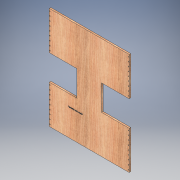
# Autodesk Inventor part: Placeholder Belly Pan
Saved by Autodesk Inventor 2018 (Build 220112000, 112)
## iProperties
Created: 2020-01-18
Part Number: Placeholder Belly Pan
Material: Wood (Birch)
Document SubType Name: Modeling
Designer: maste
Density: 0.55 g/cm^3
Appearance: Birch - Natural Polished
Author: maste
Autodesk Inventor part; units mm, degrees
ref_plane "YZ Plane" through (0, 0, 0) normal (1, 0, 0) x (0, 1, 0)
ref_plane "XZ Plane" through (0, 0, 0) normal (0, 1, 0) x (-1, 0, 0)
ref_plane "XY Plane" through (0, 0, 0) normal (0, 0, 1) x (1, 0, 0)
sketch "Sketch1" plane through (0, 0, 0) normal (0, 0, 1) x (1, 0, 0)
  line L0 (0, 0) -> (476.25, 0)
  line L1 (476.25, 0) -> (476.25, 228.6)
  line L2 (476.25, 228.6) -> (311.15, 228.6)
  line L3 (311.15, 228.6) -> (311.15, 381)
  line L4 (311.15, 381) -> (476.25, 381)
  line L5 (476.25, 381) -> (476.25, 609.6)
  line L6 (476.25, 609.6) -> (0, 609.6)
  line L7 (0, 609.6) -> (0, 381)
  line L8 (0, 381) -> (165.1, 381)
  line L9 (165.1, 381) -> (165.1, 228.6)
  line L10 (165.1, 228.6) -> (0, 228.6)
  line L11 (0, 228.6) -> (0, 0)
  dimension "d0" = 476.25
  dimension "d1" = 228.6
  dimension "d2" = 165.1
  dimension "d3" = 152.4
  dimension "d4" = 228.6
  dimension "d5" = 165.1
  constraints: 24 end point, 8 perpendicular, 7 point on line, 1 horizontal
  measures "d0" distance of L0.start L0.end
  measures "d1" distance of L0.end L1.end
  measures "d2" distance of L1.end L2.end
  measures "d3" distance of L2.end L3.end
  measures "d4" distance of L4.end L5.end
  measures "d5" distance of L7.end L8.end
extrude "Extrusion1" add sketch "Sketch1" along normal blind 9.525
sketch "Sketch2" plane through (0, 0, 9.525) normal (0, 0, 1) x (1, 0, 0)
  line L0 (0, 0) -> (3.175, 0) construction
  line L1 (0, 0) -> (476.25, 0) construction
  line L2 (3.175, 0) -> (3.175, 12.7) construction
  line L3 (3.175, 12.7) -> (3.175, 38.1) construction
  line L4 (3.175, 38.1) -> (3.175, 63.5) construction
  line L5 (3.175, 63.5) -> (3.175, 88.9) construction
  line L6 (3.175, 88.9) -> (3.175, 114.3) construction
  line L7 (3.175, 114.3) -> (3.175, 139.7) construction
  line L8 (3.175, 139.7) -> (3.175, 165.1) construction
  line L9 (3.175, 165.1) -> (3.175, 190.5) construction
  line L10 (3.175, 190.5) -> (3.175, 215.9) construction
  circle A0 centre (3.175, 12.7) radius 2.5797
  circle A1 centre (3.175, 38.1) radius 2.5797
  circle A2 centre (3.175, 63.5) radius 2.5797
  circle A3 centre (3.175, 88.9) radius 2.5797
  circle A4 centre (3.175, 114.3) radius 2.5797
  circle A5 centre (3.175, 139.7) radius 2.5797
  circle A6 centre (3.175, 165.1) radius 2.5797
  circle A7 centre (3.175, 190.5) radius 2.5797
  circle A8 centre (3.175, 215.9) radius 2.5797
  line L11 (238.125, 0) -> (238.125, 609.6) construction
  line L12 (476.25, 609.6) -> (0, 609.6) construction
  line L13 (0, 304.8) -> (476.25, 304.8) construction
  line L14 (473.075, 0) -> (473.075, 12.7) construction
  line L15 (473.075, 12.7) -> (473.075, 38.1) construction
  line L16 (473.075, 38.1) -> (473.075, 63.5) construction
  line L17 (473.075, 63.5) -> (473.075, 88.9) construction
  line L18 (473.075, 88.9) -> (473.075, 114.3) construction
  line L19 (473.075, 114.3) -> (473.075, 139.7) construction
  line L20 (473.075, 139.7) -> (473.075, 165.1) construction
  line L21 (473.075, 165.1) -> (473.075, 190.5) construction
  line L22 (473.075, 190.5) -> (473.075, 215.9) construction
  circle A9 centre (473.075, 12.7) radius 2.5797
  circle A10 centre (473.075, 38.1) radius 2.5797
  circle A11 centre (473.075, 63.5) radius 2.5797
  circle A12 centre (473.075, 88.9) radius 2.5797
  circle A13 centre (473.075, 114.3) radius 2.5797
  circle A14 centre (473.075, 139.7) radius 2.5797
  circle A15 centre (473.075, 165.1) radius 2.5797
  circle A16 centre (473.075, 190.5) radius 2.5797
  circle A17 centre (473.075, 215.9) radius 2.5797
  line L23 (0, 609.6) -> (3.175, 609.6) construction
  line L24 (0, 609.6) -> (476.25, 609.6) construction
  line L25 (3.175, 609.6) -> (3.175, 596.9) construction
  line L26 (3.175, 596.9) -> (3.175, 571.5) construction
  line L27 (3.175, 571.5) -> (3.175, 546.1) construction
  line L28 (3.175, 546.1) -> (3.175, 520.7) construction
  line L29 (3.175, 520.7) -> (3.175, 495.3) construction
  line L30 (3.175, 495.3) -> (3.175, 469.9) construction
  line L31 (3.175, 469.9) -> (3.175, 444.5) construction
  line L32 (3.175, 444.5) -> (3.175, 419.1) construction
  line L33 (3.175, 419.1) -> (3.175, 393.7) construction
  circle A18 centre (3.175, 596.9) radius 2.5797
  circle A19 centre (3.175, 571.5) radius 2.5797
  circle A20 centre (3.175, 546.1) radius 2.5797
  circle A21 centre (3.175, 520.7) radius 2.5797
  circle A22 centre (3.175, 495.3) radius 2.5797
  circle A23 centre (3.175, 469.9) radius 2.5797
  circle A24 centre (3.175, 444.5) radius 2.5797
  circle A25 centre (3.175, 419.1) radius 2.5797
  circle A26 centre (3.175, 393.7) radius 2.5797
  line L34 (473.075, 495.3) -> (473.075, 469.9) construction
  circle A27 centre (473.075, 495.3) radius 2.5797
  line L35 (473.075, 520.7) -> (473.075, 495.3) construction
  line L36 (473.075, 546.1) -> (473.075, 520.7) construction
  line L37 (473.075, 571.5) -> (473.075, 546.1) construction
  line L38 (473.075, 596.9) -> (473.075, 571.5) construction
  circle A28 centre (473.075, 596.9) radius 2.5797
  line L39 (473.075, 609.6) -> (473.075, 596.9) construction
  circle A29 centre (473.075, 520.7) radius 2.5797
  circle A30 centre (473.075, 469.9) radius 2.5797
  circle A31 centre (473.075, 444.5) radius 2.5797
  line L40 (473.075, 444.5) -> (473.075, 419.1) construction
  circle A32 centre (473.075, 419.1) radius 2.5797
  line L41 (473.075, 419.1) -> (473.075, 393.7) construction
  circle A33 centre (473.075, 393.7) radius 2.5797
  circle A34 centre (473.075, 571.5) radius 2.5797
  circle A35 centre (473.075, 546.1) radius 2.5797
  line L42 (473.075, 469.9) -> (473.075, 444.5) construction
  dimension "d8" = 3.175
  dimension "d9" = 12.7
  dimension "d10" = 25.4
  dimension "d11" = 25.4
  dimension "d12" = 25.4
  dimension "d13" = 25.4
  dimension "d14" = 25.4
  dimension "d15" = 25.4
  dimension "d16" = 25.4
  dimension "d17" = 25.4
  dimension "d18" = 5.1594
  constraints: 82 end point, 57 symmetric about line, 36 centre point, 36 coincident, 30 point on line, 2 midpoint, 2 vertical, 1 horizontal, 27 other
  measures "d8" distance of L0.start L0.end
  measures "d9" distance of L0.end L2.end
  measures "d10" distance of L2.end L3.end
  measures "d11" distance of L3.end L4.end
  measures "d12" distance of L4.end L5.end
  measures "d13" distance of L5.end L6.end
  measures "d14" distance of L6.end L7.end
  measures "d15" distance of L7.end L8.end
  measures "d16" distance of L8.end L9.end
  measures "d17" distance of L9.end L10.end
  measures "d18" diameter of A0
extrude "Extrusion2" cut sketch "Sketch2" against normal blind 82.55
sketch "Sketch3" plane through (0, 0, 9.525) normal (0, 0, 1) x (1, 0, 0)
  line L0 (113.0988, 164.0574) -> (392.0139, 164.0574) construction
  line L1 (392.0139, 164.0574) -> (392.0139, 75.3899) construction
  line L2 (392.0139, 75.3899) -> (113.0988, 75.3899) construction
  line L3 (113.0988, 75.3899) -> (113.0988, 164.0574) construction
  line L4 (117.2238, 161.3206) -> (116.957, 160.871)
  line L5 (116.957, 160.871) -> (115.6183, 161.7602)
  line L6 (115.6183, 161.7602) -> (115.6479, 160.2684)
  line L7 (115.6479, 160.2684) -> (115.1341, 160.2684)
  line L8 (115.1341, 160.2684) -> (115.1588, 161.7602)
  line L9 (115.1588, 161.7602) -> (113.83, 160.8661)
  line L10 (113.83, 160.8661) -> (113.5583, 161.3156)
  line L11 (113.5583, 161.3156) -> (115.0057, 162.1653)
  line L12 (115.0057, 162.1653) -> (113.5583, 163.0101)
  line L13 (113.5583, 163.0101) -> (113.83, 163.4596)
  line L14 (113.83, 163.4596) -> (115.1638, 162.5655)
  line L15 (115.1638, 162.5655) -> (115.1341, 164.0574)
  line L16 (115.1341, 164.0574) -> (115.6479, 164.0574)
  line L17 (115.6479, 164.0574) -> (115.6133, 162.5655)
  line L18 (115.6133, 162.5655) -> (116.957, 163.4547)
  line L19 (116.957, 163.4547) -> (117.2238, 163.0051)
  line L20 (117.2238, 163.0051) -> (115.7763, 162.1653)
  line L21 (115.7763, 162.1653) -> (117.2238, 161.3206)
  spline S0 degree 2 poles (122.065, 160.1004) (122.065, 158.9543) (120.9733, 157.6007) (120.1384, 157.6007) knots 0 0 0 1 2 2 2
  spline S1 degree 2 poles (120.1384, 157.6007) (119.7975, 157.6007) (119.2739, 157.7588) (119.0022, 157.9218) knots 0 0 0 1 2 2 2
  line L22 (119.0022, 157.9218) -> (119.0022, 156.0051)
  line L23 (119.0022, 156.0051) -> (118.2315, 156.0051)
  line L24 (118.2315, 156.0051) -> (118.2315, 162.2641)
  line L25 (118.2315, 162.2641) -> (119.0022, 162.2641)
  line L26 (119.0022, 162.2641) -> (119.0022, 161.7849)
  spline S2 degree 2 poles (119.0022, 161.7849) (119.2887, 162.0468) (119.9902, 162.3926) (120.4002, 162.3926) knots 0 0 0 1 2 2 2
  spline S3 degree 2 poles (120.4002, 162.3926) (121.1857, 162.3926) (122.065, 161.1477) (122.065, 160.1004) knots 0 0 0 1 2 2 2
  spline S4 degree 2 poles (121.2697, 160.0115) (121.2697, 160.7969) (120.7707, 161.6614) (120.2125, 161.6614) knots 0 0 0 1 2 2 2
  spline S5 degree 2 poles (120.2125, 161.6614) (119.8864, 161.6614) (119.2739, 161.37) (119.0022, 161.1427) knots 0 0 0 1 2 2 2
  line L27 (119.0022, 161.1427) -> (119.0022, 158.5443)
  spline S6 degree 2 poles (119.0022, 158.5443) (119.3035, 158.401) (119.7333, 158.2923) (120.0099, 158.2923) knots 0 0 0 1 2 2 2
  spline S7 degree 2 poles (120.0099, 158.2923) (120.6077, 158.2923) (121.2697, 159.1717) (121.2697, 160.0115) knots 0 0 0 1 2 2 2
  line L28 (125.2908, 161.4391) -> (125.2513, 161.4391)
  spline S8 degree 2 poles (125.2513, 161.4391) (125.1624, 161.4638) (124.9697, 161.4737) (124.8364, 161.4737) knots 0 0 0 1 2 2 2
  spline S9 degree 2 poles (124.8364, 161.4737) (124.5251, 161.4737) (123.9126, 161.202) (123.6359, 160.9353) knots 0 0 0 1 2 2 2
  line L29 (123.6359, 160.9353) -> (123.6359, 157.6897)
  line L30 (123.6359, 157.6897) -> (122.8653, 157.6897)
  line L31 (122.8653, 157.6897) -> (122.8653, 162.2641)
  line L32 (122.8653, 162.2641) -> (123.6359, 162.2641)
  line L33 (123.6359, 162.2641) -> (123.6359, 161.5824)
  spline S10 degree 2 poles (123.6359, 161.5824) (124.0558, 161.9578) (124.6832, 162.2641) (124.9796, 162.2641) knots 0 0 0 1 2 2 2
  spline S11 degree 2 poles (124.9796, 162.2641) (125.0982, 162.2641) (125.2167, 162.2542) (125.2908, 162.2394) knots 0 0 0 1 2 2 2
  line L34 (125.2908, 162.2394) -> (125.2908, 161.4391)
  spline S12 degree 2 poles (129.648, 159.9769) (129.648, 158.8209) (128.5364, 157.5612) (127.6077, 157.5612) knots 0 0 0 1 2 2 2
  spline S13 degree 2 poles (127.6077, 157.5612) (126.6543, 157.5612) (125.5625, 158.8604) (125.5625, 159.9769) knots 0 0 0 1 2 2 2
  spline S14 degree 2 poles (125.5625, 159.9769) (125.5625, 161.123) (126.6889, 162.3926) (127.6077, 162.3926) knots 0 0 0 1 2 2 2
  spline S15 degree 2 poles (127.6077, 162.3926) (128.5364, 162.3926) (129.648, 161.1279) (129.648, 159.9769) knots 0 0 0 1 2 2 2
  spline S16 degree 2 poles (128.8526, 159.9769) (128.8526, 160.8661) (128.2055, 161.7306) (127.6077, 161.7306) knots 0 0 0 1 2 2 2
  spline S17 degree 2 poles (127.6077, 161.7306) (127.01, 161.7306) (126.3579, 160.8661) (126.3579, 159.9769) knots 0 0 0 1 2 2 2
  spline S18 degree 2 poles (126.3579, 159.9769) (126.3579, 159.1124) (127.01, 158.2232) (127.6077, 158.2232) knots 0 0 0 1 2 2 2
  spline S19 degree 2 poles (127.6077, 158.2232) (128.2005, 158.2232) (128.8526, 159.0976) (128.8526, 159.9769) knots 0 0 0 1 2 2 2
  spline S20 degree 2 poles (134.2718, 160.051) (134.2718, 158.9296) (133.185, 157.5612) (132.365, 157.5612) knots 0 0 0 1 2 2 2
  spline S21 degree 2 poles (132.365, 157.5612) (131.9945, 157.5612) (131.4659, 157.744) (131.209, 157.9021) knots 0 0 0 1 2 2 2
  line L35 (131.209, 157.9021) -> (131.1596, 157.6897)
  line L36 (131.1596, 157.6897) -> (130.4384, 157.6897)
  line L37 (130.4384, 157.6897) -> (130.4384, 164.0574)
  line L38 (130.4384, 164.0574) -> (131.209, 164.0574)
  line L39 (131.209, 164.0574) -> (131.209, 161.7849)
  spline S22 degree 2 poles (131.209, 161.7849) (131.5005, 162.0468) (132.1772, 162.3926) (132.607, 162.3926) knots 0 0 0 1 2 2 2
  spline S23 degree 2 poles (132.607, 162.3926) (133.3826, 162.3926) (134.2718, 161.1526) (134.2718, 160.051) knots 0 0 0 1 2 2 2
  spline S24 degree 2 poles (133.4765, 159.9917) (133.4765, 160.8118) (132.9775, 161.6614) (132.4243, 161.6614) knots 0 0 0 1 2 2 2
  spline S25 degree 2 poles (132.4243, 161.6614) (132.113, 161.6614) (131.4708, 161.365) (131.209, 161.1378) knots 0 0 0 1 2 2 2
  line L40 (131.209, 161.1378) -> (131.209, 158.5146)
  spline S26 degree 2 poles (131.209, 158.5146) (131.5005, 158.3714) (131.95, 158.2528) (132.2168, 158.2528) knots 0 0 0 1 2 2 2
  spline S27 degree 2 poles (132.2168, 158.2528) (132.8046, 158.2528) (133.4765, 159.0877) (133.4765, 159.9917) knots 0 0 0 1 2 2 2
  spline S28 degree 2 poles (137.6212, 158.1738) (137.5273, 158.1046) (137.2111, 157.8576) (137.0629, 157.7835) knots 0 0 0 1 2 2 2
  spline S29 degree 2 poles (137.0629, 157.7835) (136.8604, 157.6748) (136.48, 157.5612) (136.1342, 157.5612) knots 0 0 0 1 2 2 2
  spline S30 degree 2 poles (136.1342, 157.5612) (135.8526, 157.5612) (135.3438, 157.7736) (135.1511, 157.9663) knots 0 0 0 1 2 2 2
  spline S31 degree 2 poles (135.1511, 157.9663) (134.9684, 158.154) (134.7461, 158.7073) (134.7461, 159.0136) knots 0 0 0 1 2 2 2
  spline S32 degree 2 poles (134.7461, 159.0136) (134.7461, 159.4878) (135.1462, 160.1597) (135.5809, 160.3523) knots 0 0 0 1 2 2 2
  spline S33 degree 2 poles (135.5809, 160.3523) (135.9663, 160.5302) (137.0135, 160.6636) (137.6212, 160.6981) knots 0 0 0 1 2 2 2
  line L41 (137.6212, 160.6981) -> (137.6212, 160.8463)
  spline S34 degree 2 poles (137.6212, 160.8463) (137.6212, 161.1131) (137.4581, 161.4441) (137.3099, 161.5379) knots 0 0 0 1 2 2 2
  spline S35 degree 2 poles (137.3099, 161.5379) (137.1617, 161.6318) (136.7369, 161.6911) (136.5097, 161.6911) knots 0 0 0 1 2 2 2
  spline S36 degree 2 poles (136.5097, 161.6911) (136.2429, 161.6911) (135.5217, 161.533) (135.161, 161.3799) knots 0 0 0 1 2 2 2
  line L42 (135.161, 161.3799) -> (135.1166, 161.3799)
  line L43 (135.1166, 161.3799) -> (135.1166, 162.1653)
  spline S37 degree 2 poles (135.1166, 162.1653) (135.329, 162.2246) (136.1243, 162.3728) (136.5146, 162.3728) knots 0 0 0 1 2 2 2
  spline S38 degree 2 poles (136.5146, 162.3728) (136.9888, 162.3728) (137.636, 162.2246) (137.8929, 162.0319) knots 0 0 0 1 2 2 2
  spline S39 degree 2 poles (137.8929, 162.0319) (138.1448, 161.8442) (138.3918, 161.2465) (138.3918, 160.8167) knots 0 0 0 1 2 2 2
  line L44 (138.3918, 160.8167) -> (138.3918, 157.6897)
  line L45 (138.3918, 157.6897) -> (137.6212, 157.6897)
  line L46 (137.6212, 157.6897) -> (137.6212, 158.1738)
  line L47 (137.6212, 158.816) -> (137.6212, 160.0856)
  spline S40 degree 2 poles (137.6212, 160.0856) (137.3445, 160.0609) (136.5097, 159.9769) (136.2478, 159.8978) knots 0 0 0 1 2 2 2
  spline S41 degree 2 poles (136.2478, 159.8978) (135.9416, 159.804) (135.5414, 159.4137) (135.5414, 159.0679) knots 0 0 0 1 2 2 2
  spline S42 degree 2 poles (135.5414, 159.0679) (135.5414, 158.6727) (135.986, 158.2726) (136.4109, 158.2726) knots 0 0 0 1 2 2 2
  spline S43 degree 2 poles (136.4109, 158.2726) (136.7715, 158.2726) (137.3643, 158.5838) (137.6212, 158.816) knots 0 0 0 1 2 2 2
  spline S44 degree 2 poles (143.3071, 160.051) (143.3071, 158.9296) (142.2203, 157.5612) (141.4003, 157.5612) knots 0 0 0 1 2 2 2
  spline S45 degree 2 poles (141.4003, 157.5612) (141.0298, 157.5612) (140.5012, 157.744) (140.2443, 157.9021) knots 0 0 0 1 2 2 2
  line L48 (140.2443, 157.9021) -> (140.1949, 157.6897)
  line L49 (140.1949, 157.6897) -> (139.4737, 157.6897)
  line L50 (139.4737, 157.6897) -> (139.4737, 164.0574)
  line L51 (139.4737, 164.0574) -> (140.2443, 164.0574)
  line L52 (140.2443, 164.0574) -> (140.2443, 161.7849)
  spline S46 degree 2 poles (140.2443, 161.7849) (140.5358, 162.0468) (141.2126, 162.3926) (141.6424, 162.3926) knots 0 0 0 1 2 2 2
  spline S47 degree 2 poles (141.6424, 162.3926) (142.4179, 162.3926) (143.3071, 161.1526) (143.3071, 160.051) knots 0 0 0 1 2 2 2
  spline S48 degree 2 poles (142.5118, 159.9917) (142.5118, 160.8118) (142.0129, 161.6614) (141.4596, 161.6614) knots 0 0 0 1 2 2 2
  spline S49 degree 2 poles (141.4596, 161.6614) (141.1483, 161.6614) (140.5061, 161.365) (140.2443, 161.1378) knots 0 0 0 1 2 2 2
  line L53 (140.2443, 161.1378) -> (140.2443, 158.5146)
  spline S50 degree 2 poles (140.2443, 158.5146) (140.5358, 158.3714) (140.9853, 158.2528) (141.2521, 158.2528) knots 0 0 0 1 2 2 2
  spline S51 degree 2 poles (141.2521, 158.2528) (141.84, 158.2528) (142.5118, 159.0877) (142.5118, 159.9917) knots 0 0 0 1 2 2 2
  line L54 (144.8929, 157.6897) -> (144.1222, 157.6897)
  line L55 (144.1222, 157.6897) -> (144.1222, 164.0574)
  line L56 (144.1222, 164.0574) -> (144.8929, 164.0574)
  line L57 (144.8929, 164.0574) -> (144.8929, 157.6897)
  line L58 (149.6156, 162.2641) -> (147.1554, 156.0051)
  line L59 (147.1554, 156.0051) -> (146.3304, 156.0051)
  line L60 (146.3304, 156.0051) -> (147.1505, 157.912)
  line L61 (147.1505, 157.912) -> (145.4906, 162.2641)
  line L62 (145.4906, 162.2641) -> (146.3206, 162.2641)
  line L63 (146.3206, 162.2641) -> (147.5704, 158.8753)
  line L64 (147.5704, 158.8753) -> (148.8153, 162.2641)
  line L65 (148.8153, 162.2641) -> (149.6156, 162.2641)
  line L66 (156.4081, 157.6897) -> (155.6375, 157.6897)
  line L67 (155.6375, 157.6897) -> (155.6375, 160.298)
  spline S52 degree 2 poles (155.6375, 160.298) (155.6375, 160.6142) (155.5782, 161.1576) (155.4893, 161.3206) knots 0 0 0 1 2 2 2
  spline S53 degree 2 poles (155.4893, 161.3206) (155.3954, 161.4935) (155.0595, 161.6614) (154.773, 161.6614) knots 0 0 0 1 2 2 2
  spline S54 degree 2 poles (154.773, 161.6614) (154.4864, 161.6614) (153.8788, 161.3552) (153.5873, 161.1082) knots 0 0 0 1 2 2 2
  line L68 (153.5873, 161.1082) -> (153.5873, 157.6897)
  line L69 (153.5873, 157.6897) -> (152.8167, 157.6897)
  line L70 (152.8167, 157.6897) -> (152.8167, 162.2641)
  line L71 (152.8167, 162.2641) -> (153.5873, 162.2641)
  line L72 (153.5873, 162.2641) -> (153.5873, 161.7553)
  spline S55 degree 2 poles (153.5873, 161.7553) (153.9332, 162.0665) (154.6001, 162.3926) (154.9755, 162.3926) knots 0 0 0 1 2 2 2
  spline S56 degree 2 poles (154.9755, 162.3926) (155.6473, 162.3926) (156.4081, 161.5034) (156.4081, 160.6586) knots 0 0 0 1 2 2 2
  line L73 (156.4081, 160.6586) -> (156.4081, 157.6897)
  spline S57 degree 2 poles (161.2493, 159.9769) (161.2493, 158.8209) (160.1378, 157.5612) (159.2091, 157.5612) knots 0 0 0 1 2 2 2
  spline S58 degree 2 poles (159.2091, 157.5612) (158.2557, 157.5612) (157.1639, 158.8604) (157.1639, 159.9769) knots 0 0 0 1 2 2 2
  spline S59 degree 2 poles (157.1639, 159.9769) (157.1639, 161.123) (158.2903, 162.3926) (159.2091, 162.3926) knots 0 0 0 1 2 2 2
  spline S60 degree 2 poles (159.2091, 162.3926) (160.1378, 162.3926) (161.2493, 161.1279) (161.2493, 159.9769) knots 0 0 0 1 2 2 2
  spline S61 degree 2 poles (160.454, 159.9769) (160.454, 160.8661) (159.8069, 161.7306) (159.2091, 161.7306) knots 0 0 0 1 2 2 2
  spline S62 degree 2 poles (159.2091, 161.7306) (158.6114, 161.7306) (157.9593, 160.8661) (157.9593, 159.9769) knots 0 0 0 1 2 2 2
  spline S63 degree 2 poles (157.9593, 159.9769) (157.9593, 159.1124) (158.6114, 158.2232) (159.2091, 158.2232) knots 0 0 0 1 2 2 2
  spline S64 degree 2 poles (159.2091, 158.2232) (159.8019, 158.2232) (160.454, 159.0976) (160.454, 159.9769) knots 0 0 0 1 2 2 2
  spline S65 degree 2 poles (163.423, 157.6007) (162.7956, 157.6007) (162.0891, 158.317) (162.0891, 159.0926) knots 0 0 0 1 2 2 2
  line L74 (162.0891, 159.0926) -> (162.0891, 161.6269)
  line L75 (162.0891, 161.6269) -> (161.5704, 161.6269)
  line L76 (161.5704, 161.6269) -> (161.5704, 162.2641)
  line L77 (161.5704, 162.2641) -> (162.0891, 162.2641)
  line L78 (162.0891, 162.2641) -> (162.0891, 163.5782)
  line L79 (162.0891, 163.5782) -> (162.8598, 163.5782)
  line L80 (162.8598, 163.5782) -> (162.8598, 162.2641)
  line L81 (162.8598, 162.2641) -> (164.2776, 162.2641)
  line L82 (164.2776, 162.2641) -> (164.2776, 161.6269)
  line L83 (164.2776, 161.6269) -> (162.8598, 161.6269)
  line L84 (162.8598, 161.6269) -> (162.8598, 159.4483)
  spline S66 degree 2 poles (162.8598, 159.4483) (162.8598, 159.1025) (162.8845, 158.7221) (162.9685, 158.5591) knots 0 0 0 1 2 2 2
  spline S67 degree 2 poles (162.9685, 158.5591) (163.0376, 158.4158) (163.3489, 158.2726) (163.6156, 158.2726) knots 0 0 0 1 2 2 2
  spline S68 degree 2 poles (163.6156, 158.2726) (163.8033, 158.2726) (164.1541, 158.3862) (164.2331, 158.4208) knots 0 0 0 1 2 2 2
  line L85 (164.2331, 158.4208) -> (164.2776, 158.4208)
  line L86 (164.2776, 158.4208) -> (164.2776, 157.7292)
  spline S69 degree 2 poles (164.2776, 157.7292) (164.0602, 157.6699) (163.6156, 157.6007) (163.423, 157.6007) knots 0 0 0 1 2 2 2
  spline S70 degree 2 poles (168.8471, 157.6007) (168.2197, 157.6007) (167.5133, 158.317) (167.5133, 159.0926) knots 0 0 0 1 2 2 2
  line L87 (167.5133, 159.0926) -> (167.5133, 161.6269)
  line L88 (167.5133, 161.6269) -> (166.9946, 161.6269)
  line L89 (166.9946, 161.6269) -> (166.9946, 162.2641)
  line L90 (166.9946, 162.2641) -> (167.5133, 162.2641)
  line L91 (167.5133, 162.2641) -> (167.5133, 163.5782)
  line L92 (167.5133, 163.5782) -> (168.2839, 163.5782)
  line L93 (168.2839, 163.5782) -> (168.2839, 162.2641)
  line L94 (168.2839, 162.2641) -> (169.7017, 162.2641)
  line L95 (169.7017, 162.2641) -> (169.7017, 161.6269)
  line L96 (169.7017, 161.6269) -> (168.2839, 161.6269)
  line L97 (168.2839, 161.6269) -> (168.2839, 159.4483)
  spline S71 degree 2 poles (168.2839, 159.4483) (168.2839, 159.1025) (168.3086, 158.7221) (168.3926, 158.5591) knots 0 0 0 1 2 2 2
  spline S72 degree 2 poles (168.3926, 158.5591) (168.4618, 158.4158) (168.773, 158.2726) (169.0398, 158.2726) knots 0 0 0 1 2 2 2
  spline S73 degree 2 poles (169.0398, 158.2726) (169.2275, 158.2726) (169.5782, 158.3862) (169.6573, 158.4208) knots 0 0 0 1 2 2 2
  line L98 (169.6573, 158.4208) -> (169.7017, 158.4208)
  line L99 (169.7017, 158.4208) -> (169.7017, 157.7292)
  spline S74 degree 2 poles (169.7017, 157.7292) (169.4844, 157.6699) (169.0398, 157.6007) (168.8471, 157.6007) knots 0 0 0 1 2 2 2
  spline S75 degree 2 poles (174.0292, 159.9769) (174.0292, 158.8209) (172.9177, 157.5612) (171.989, 157.5612) knots 0 0 0 1 2 2 2
  spline S76 degree 2 poles (171.989, 157.5612) (171.0355, 157.5612) (169.9438, 158.8604) (169.9438, 159.9769) knots 0 0 0 1 2 2 2
  spline S77 degree 2 poles (169.9438, 159.9769) (169.9438, 161.123) (171.0701, 162.3926) (171.989, 162.3926) knots 0 0 0 1 2 2 2
  spline S78 degree 2 poles (171.989, 162.3926) (172.9177, 162.3926) (174.0292, 161.1279) (174.0292, 159.9769) knots 0 0 0 1 2 2 2
  spline S79 degree 2 poles (173.2339, 159.9769) (173.2339, 160.8661) (172.5867, 161.7306) (171.989, 161.7306) knots 0 0 0 1 2 2 2
  spline S80 degree 2 poles (171.989, 161.7306) (171.3912, 161.7306) (170.7391, 160.8661) (170.7391, 159.9769) knots 0 0 0 1 2 2 2
  spline S81 degree 2 poles (170.7391, 159.9769) (170.7391, 159.1124) (171.3912, 158.2232) (171.989, 158.2232) knots 0 0 0 1 2 2 2
  spline S82 degree 2 poles (171.989, 158.2232) (172.5818, 158.2232) (173.2339, 159.0976) (173.2339, 159.9769) knots 0 0 0 1 2 2 2
  spline S83 degree 2 poles (178.6728, 157.581) (178.2134, 157.581) (177.4181, 157.828) (177.1562, 157.9663) knots 0 0 0 1 2 2 2
  line L100 (177.1562, 157.9663) -> (177.1562, 158.8308)
  line L101 (177.1562, 158.8308) -> (177.1958, 158.8308)
  spline S84 degree 2 poles (177.1958, 158.8308) (177.2946, 158.7518) (177.5613, 158.564) (177.7836, 158.4603) knots 0 0 0 1 2 2 2
  spline S85 degree 2 poles (177.7836, 158.4603) (177.9763, 158.3664) (178.4505, 158.2281) (178.7025, 158.2281) knots 0 0 0 1 2 2 2
  spline S86 degree 2 poles (178.7025, 158.2281) (178.8853, 158.2281) (179.3052, 158.3121) (179.404, 158.3813) knots 0 0 0 1 2 2 2
  spline S87 degree 2 poles (179.404, 158.3813) (179.5472, 158.4751) (179.6757, 158.6875) (179.6757, 158.9049) knots 0 0 0 1 2 2 2
  spline S88 degree 2 poles (179.6757, 158.9049) (179.6757, 159.1766) (179.3793, 159.4582) (178.9989, 159.552) knots 0 0 0 1 2 2 2
  spline S89 degree 2 poles (178.9989, 159.552) (178.8507, 159.5866) (178.3764, 159.6854) (178.1739, 159.7398) knots 0 0 0 1 2 2 2
  spline S90 degree 2 poles (178.1739, 159.7398) (177.6502, 159.8929) (177.176, 160.5252) (177.176, 160.9748) knots 0 0 0 1 2 2 2
  spline S91 degree 2 poles (177.176, 160.9748) (177.176, 161.5972) (178.1097, 162.3728) (178.8803, 162.3728) knots 0 0 0 1 2 2 2
  spline S92 degree 2 poles (178.8803, 162.3728) (179.2607, 162.3728) (180.0313, 162.1851) (180.2932, 162.0418) knots 0 0 0 1 2 2 2
  line L102 (180.2932, 162.0418) -> (180.2932, 161.2168)
  line L103 (180.2932, 161.2168) -> (180.2536, 161.2168)
  spline S93 degree 2 poles (180.2536, 161.2168) (179.9572, 161.454) (179.236, 161.7257) (178.8655, 161.7257) knots 0 0 0 1 2 2 2
  spline S94 degree 2 poles (178.8655, 161.7257) (178.4851, 161.7257) (177.9615, 161.4046) (177.9615, 161.0835) knots 0 0 0 1 2 2 2
  spline S95 degree 2 poles (177.9615, 161.0835) (177.9615, 160.792) (178.2727, 160.5104) (178.6185, 160.4215) knots 0 0 0 1 2 2 2
  spline S96 degree 2 poles (178.6185, 160.4215) (178.7865, 160.377) (179.2113, 160.2881) (179.4435, 160.2338) knots 0 0 0 1 2 2 2
  spline S97 degree 2 poles (179.4435, 160.2338) (179.9474, 160.1053) (180.4611, 159.5175) (180.4611, 159.0086) knots 0 0 0 1 2 2 2
  spline S98 degree 2 poles (180.4611, 159.0086) (180.4611, 158.7122) (180.2289, 158.1886) (180.0017, 157.9959) knots 0 0 0 1 2 2 2
  spline S99 degree 2 poles (180.0017, 157.9959) (179.7596, 157.7934) (179.1421, 157.581) (178.6728, 157.581) knots 0 0 0 1 2 2 2
  spline S100 degree 2 poles (182.9954, 157.5859) (182.5211, 157.5859) (181.7357, 157.8774) (181.4541, 158.1738) knots 0 0 0 1 2 2 2
  spline S101 degree 2 poles (181.4541, 158.1738) (181.1725, 158.4652) (180.8613, 159.3643) (180.8613, 159.967) knots 0 0 0 1 2 2 2
  spline S102 degree 2 poles (180.8613, 159.967) (180.8613, 160.5697) (181.1824, 161.449) (181.4541, 161.7454) knots 0 0 0 1 2 2 2
  spline S103 degree 2 poles (181.4541, 161.7454) (181.7258, 162.0468) (182.531, 162.3679) (182.9954, 162.3679) knots 0 0 0 1 2 2 2
  spline S104 degree 2 poles (182.9954, 162.3679) (183.3708, 162.3679) (184.0723, 162.1554) (184.344, 162.0171) knots 0 0 0 1 2 2 2
  line L104 (184.344, 162.0171) -> (184.344, 161.1526)
  line L105 (184.344, 161.1526) -> (184.2995, 161.1526)
  spline S105 degree 2 poles (184.2995, 161.1526) (184.2156, 161.2218) (183.9587, 161.3996) (183.7759, 161.4935) knots 0 0 0 1 2 2 2
  spline S106 degree 2 poles (183.7759, 161.4935) (183.6129, 161.5725) (183.1781, 161.696) (182.9805, 161.696) knots 0 0 0 1 2 2 2
  spline S107 degree 2 poles (182.9805, 161.696) (182.3828, 161.696) (181.6566, 160.792) (181.6566, 159.967) knots 0 0 0 1 2 2 2
  spline S108 degree 2 poles (181.6566, 159.967) (181.6566, 159.1618) (182.3581, 158.2578) (182.9805, 158.2578) knots 0 0 0 1 2 2 2
  spline S109 degree 2 poles (182.9805, 158.2578) (183.356, 158.2578) (184.0377, 158.569) (184.2995, 158.811) knots 0 0 0 1 2 2 2
  line L106 (184.2995, 158.811) -> (184.344, 158.811)
  line L107 (184.344, 158.811) -> (184.344, 157.9465)
  spline S110 degree 2 poles (184.344, 157.9465) (184.2304, 157.8922) (183.8846, 157.7391) (183.7462, 157.7045) knots 0 0 0 1 2 2 2
  spline S111 degree 2 poles (183.7462, 157.7045) (183.5486, 157.6452) (183.2374, 157.5859) (182.9954, 157.5859) knots 0 0 0 1 2 2 2
  spline S112 degree 2 poles (187.5945, 158.1738) (187.5007, 158.1046) (187.1845, 157.8576) (187.0363, 157.7835) knots 0 0 0 1 2 2 2
  spline S113 degree 2 poles (187.0363, 157.7835) (186.8338, 157.6748) (186.4534, 157.5612) (186.1076, 157.5612) knots 0 0 0 1 2 2 2
  spline S114 degree 2 poles (186.1076, 157.5612) (185.826, 157.5612) (185.3172, 157.7736) (185.1245, 157.9663) knots 0 0 0 1 2 2 2
  spline S115 degree 2 poles (185.1245, 157.9663) (184.9417, 158.154) (184.7194, 158.7073) (184.7194, 159.0136) knots 0 0 0 1 2 2 2
  spline S116 degree 2 poles (184.7194, 159.0136) (184.7194, 159.4878) (185.1196, 160.1597) (185.5543, 160.3523) knots 0 0 0 1 2 2 2
  spline S117 degree 2 poles (185.5543, 160.3523) (185.9396, 160.5302) (186.9869, 160.6636) (187.5945, 160.6981) knots 0 0 0 1 2 2 2
  line L108 (187.5945, 160.6981) -> (187.5945, 160.8463)
  spline S118 degree 2 poles (187.5945, 160.8463) (187.5945, 161.1131) (187.4315, 161.4441) (187.2833, 161.5379) knots 0 0 0 1 2 2 2
  spline S119 degree 2 poles (187.2833, 161.5379) (187.1351, 161.6318) (186.7103, 161.6911) (186.483, 161.6911) knots 0 0 0 1 2 2 2
  spline S120 degree 2 poles (186.483, 161.6911) (186.2163, 161.6911) (185.495, 161.533) (185.1344, 161.3799) knots 0 0 0 1 2 2 2
  line L109 (185.1344, 161.3799) -> (185.0899, 161.3799)
  line L110 (185.0899, 161.3799) -> (185.0899, 162.1653)
  spline S121 degree 2 poles (185.0899, 162.1653) (185.3024, 162.2246) (186.0977, 162.3728) (186.488, 162.3728) knots 0 0 0 1 2 2 2
  spline S122 degree 2 poles (186.488, 162.3728) (186.9622, 162.3728) (187.6094, 162.2246) (187.8662, 162.0319) knots 0 0 0 1 2 2 2
  spline S123 degree 2 poles (187.8662, 162.0319) (188.1182, 161.8442) (188.3652, 161.2465) (188.3652, 160.8167) knots 0 0 0 1 2 2 2
  line L111 (188.3652, 160.8167) -> (188.3652, 157.6897)
  line L112 (188.3652, 157.6897) -> (187.5945, 157.6897)
  line L113 (187.5945, 157.6897) -> (187.5945, 158.1738)
  line L114 (187.5945, 158.816) -> (187.5945, 160.0856)
  spline S124 degree 2 poles (187.5945, 160.0856) (187.3179, 160.0609) (186.483, 159.9769) (186.2212, 159.8978) knots 0 0 0 1 2 2 2
  spline S125 degree 2 poles (186.2212, 159.8978) (185.9149, 159.804) (185.5148, 159.4137) (185.5148, 159.0679) knots 0 0 0 1 2 2 2
  spline S126 degree 2 poles (185.5148, 159.0679) (185.5148, 158.6727) (185.9594, 158.2726) (186.3842, 158.2726) knots 0 0 0 1 2 2 2
  spline S127 degree 2 poles (186.3842, 158.2726) (186.7448, 158.2726) (187.3377, 158.5838) (187.5945, 158.816) knots 0 0 0 1 2 2 2
  line L115 (190.2325, 157.6897) -> (189.4619, 157.6897)
  line L116 (189.4619, 157.6897) -> (189.4619, 164.0574)
  line L117 (189.4619, 164.0574) -> (190.2325, 164.0574)
  line L118 (190.2325, 164.0574) -> (190.2325, 157.6897)
  spline S128 degree 2 poles (193.3497, 157.5859) (192.253, 157.5859) (191.0476, 158.816) (191.0476, 159.9522) knots 0 0 0 1 2 2 2
  spline S129 degree 2 poles (191.0476, 159.9522) (191.0476, 161.0686) (192.2184, 162.3926) (193.162, 162.3926) knots 0 0 0 1 2 2 2
  spline S130 degree 2 poles (193.162, 162.3926) (193.5868, 162.3926) (194.2438, 162.1456) (194.4859, 161.8837) knots 0 0 0 1 2 2 2
  spline S131 degree 2 poles (194.4859, 161.8837) (194.7329, 161.6219) (194.9947, 160.8661) (194.9947, 160.3178) knots 0 0 0 1 2 2 2
  line L119 (194.9947, 160.3178) -> (194.9947, 159.8978)
  line L120 (194.9947, 159.8978) -> (191.8281, 159.8978)
  spline S132 degree 2 poles (191.8281, 159.8978) (191.8281, 159.1025) (192.6284, 158.2578) (193.3398, 158.2578) knots 0 0 0 1 2 2 2
  spline S133 degree 2 poles (193.3398, 158.2578) (193.5917, 158.2578) (194.0808, 158.3714) (194.2784, 158.4603) knots 0 0 0 1 2 2 2
  spline S134 degree 2 poles (194.2784, 158.4603) (194.4859, 158.5591) (194.7724, 158.732) (194.8663, 158.811) knots 0 0 0 1 2 2 2
  line L121 (194.8663, 158.811) -> (194.9107, 158.811)
  line L122 (194.9107, 158.811) -> (194.9107, 157.9712)
  spline S135 degree 2 poles (194.9107, 157.9712) (194.7773, 157.9169) (194.3723, 157.7588) (194.2142, 157.7144) knots 0 0 0 1 2 2 2
  spline S136 degree 2 poles (194.2142, 157.7144) (193.9919, 157.6501) (193.6263, 157.5859) (193.3497, 157.5859) knots 0 0 0 1 2 2 2
  spline S137 degree 2 poles (194.2438, 160.4857) (194.2339, 160.7969) (194.1055, 161.2514) (193.982, 161.4046) knots 0 0 0 1 2 2 2
  spline S138 degree 2 poles (193.982, 161.4046) (193.8486, 161.5775) (193.4287, 161.7602) (193.1175, 161.7602) knots 0 0 0 1 2 2 2
  spline S139 degree 2 poles (193.1175, 161.7602) (192.8112, 161.7602) (192.3814, 161.5775) (192.2036, 161.3996) knots 0 0 0 1 2 2 2
  spline S140 degree 2 poles (192.2036, 161.3996) (192.0307, 161.2168) (191.8528, 160.7772) (191.8281, 160.4857) knots 0 0 0 1 2 2 2
  line L123 (191.8281, 160.4857) -> (194.2438, 160.4857)
  line L124 (199.3419, 161.3206) -> (199.0752, 160.871)
  line L125 (199.0752, 160.871) -> (197.7364, 161.7602)
  line L126 (197.7364, 161.7602) -> (197.7661, 160.2684)
  line L127 (197.7661, 160.2684) -> (197.2523, 160.2684)
  line L128 (197.2523, 160.2684) -> (197.277, 161.7602)
  line L129 (197.277, 161.7602) -> (195.9481, 160.8661)
  line L130 (195.9481, 160.8661) -> (195.6764, 161.3156)
  line L131 (195.6764, 161.3156) -> (197.1239, 162.1653)
  line L132 (197.1239, 162.1653) -> (195.6764, 163.0101)
  line L133 (195.6764, 163.0101) -> (195.9481, 163.4596)
  line L134 (195.9481, 163.4596) -> (197.2819, 162.5655)
  line L135 (197.2819, 162.5655) -> (197.2523, 164.0574)
  line L136 (197.2523, 164.0574) -> (197.7661, 164.0574)
  line L137 (197.7661, 164.0574) -> (197.7315, 162.5655)
  line L138 (197.7315, 162.5655) -> (199.0752, 163.4547)
  line L139 (199.0752, 163.4547) -> (199.3419, 163.0051)
  line L140 (199.3419, 163.0051) -> (197.8945, 162.1653)
  line L141 (197.8945, 162.1653) -> (199.3419, 161.3206)
  point P0 (0, 0)
  constraints: 2 other
extrude "Extrusion3" cut sketch "Sketch3" against normal blind 25.4
body "Solid1"
